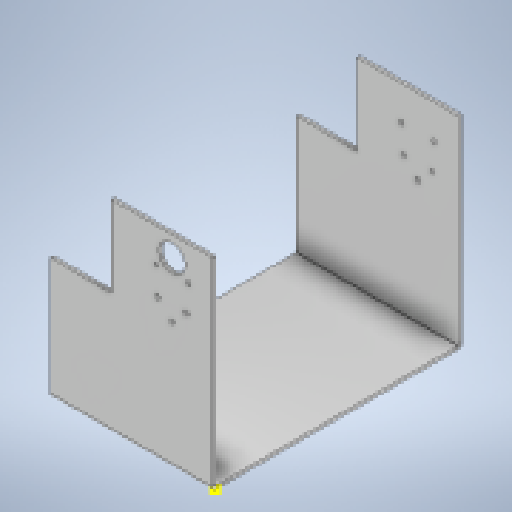
# Autodesk Inventor part: body_main_frame
Saved by Autodesk Inventor 2025.2 (Build 292293000, 293)
## iProperties
Created: 2025-05-07
Part Number: body_main_frame
Material: Aluminum 6061-AHC
Document SubType Name: Sheet Metal
Designer: chris
Density: 2.7 g/cm^3
Sheet Metal Rule: Default_mm
Appearance: Aluminum - Dark
Author: chris
Autodesk Inventor part; units mm, degrees
ref_plane "YZ Plane" through (0, 0, 0) normal (1, 0, 0) x (0, 1, 0)
ref_plane "XZ Plane" through (0, 0, 0) normal (0, 1, 0) x (-1, 0, 0)
ref_plane "XY Plane" through (0, 0, 0) normal (0, 0, 1) x (1, 0, 0)
sketch "Sketch1" plane through (0, 0, 0) normal (0, 1, 0) x (-1, 0, 0)
  line L0 (0, 0) -> (80, 0)
  line L1 (80, 0) -> (80, 120)
  line L2 (80, 120) -> (0, 120)
  line L3 (0, 120) -> (0, 0)
  dimension "d0" = 80
  dimension "d1" = 120
  measures "d0" distance of L2.end L1.end
  measures "d1" distance of L0.end L1.end
extrude "Plate1" add sketch "Sketch1" along normal blind 1.5
sketch "Sketch2" plane through (0, 0, 121.5) normal (0, 0, -1) x (-1, 0, 0)
  line L0 (80, 0) -> (0, 0)
  line L1 (0, 0) -> (0, 100)
  line L2 (0, 100) -> (80, 100)
  line L3 (80, 100) -> (80, 0)
  constraints: 8 end point
edge flange "Flange1" height 100 angle 90 thickness 1.5 bend radius 0.31 thickness toward (0, 0, -1) relief tear relief width 1.5 relief depth 0.75 edges at (-40, 1.5, 120) wall of the first edge with corners at (-80, 0, 121.5) (0, 0, 121.5) (0, 100, 121.5) (-80, 100, 121.5)
bend "Bend1"
corner "Corner1"
sketch "Sketch3" plane through (-80, 0, -1.5) normal (0, 0, 1) x (1, 0, 0)
  line L0 (80, 0) -> (0, 0)
  line L1 (0, 0) -> (0, 100)
  line L2 (0, 100) -> (80, 100)
  line L3 (80, 100) -> (80, 0)
  constraints: 6 end point, 1 horizontal, 1 perpendicular, 1 vertical
edge flange "Flange2" height 100 angle 90 thickness 1.5 bend radius 0.31 thickness toward (0, 0, 1) relief tear relief width 1.5 relief depth 0.75 edges at (-40, 1.5, 0) wall of the first edge with corners at (0, 0, -1.5) (-80, 0, -1.5) (-80, 100, -1.5) (0, 100, -1.5)
bend "Bend2"
corner "Corner2"
sketch "Sketch4" plane through (0, 100, -1.5) normal (0, 0, -1) x (-1, 0, 0)
  line L0 (56, -40) -> (80, -40)
  line L1 (80, -40) -> (80, 0)
  line L2 (80, 0) -> (56, 0)
  line L3 (56, 0) -> (56, -40)
  line L4 (80, 0) -> (80, -98.19) projected
  line L5 (0, 0) -> (80, 0) projected
  point P0 (0, -100)
  dimension "d23" = 24
  dimension "d24" = 40
  constraints: 8 end point, 2 collinear, 2 parallel, 1 horizontal, 1 perpendicular
  measures "d23" distance of L0.start L0.end
  measures "d24" distance of L2.end L0.start
extrude "Cut1" cut sketch "Sketch4" against normal blind 1.5
sketch "Sketch5" plane through (0, 100, 120) normal (0, 0, -1) x (-1, 0, 0)
  point P0 (0, -100)
sketch "Sketch6" plane through (-80, 100, 121.5) normal (0, 0, 1) x (1, 0, 0)
  line L0 (24, 0) -> (0, 0)
  line L1 (0, 0) -> (0, -40)
  line L2 (0, -40) -> (24, -40)
  line L3 (24, -40) -> (24, 0)
  line L4 (0, -98.19) -> (0, 0) projected
  line L5 (0, 0) -> (80, 0) projected
  point P0 (80, -100)
  dimension "d27" = 40
  dimension "d28" = 24
  constraints: 8 end point, 2 collinear, 2 parallel, 1 horizontal, 1 perpendicular
  measures "d27" distance of L2.end L0.start
  measures "d28" distance of L1.end L2.end
extrude "Cut2" cut sketch "Sketch6" against normal blind 1.5
sketch "Sketch7" plane through (0, 1.81, -1.5) normal (0, 0, -1) x (-1, 0, 0)
  circle A0 centre (17.93, 60.77) radius 0.7835 projected
  circle A1 centre (10.93, 68.07) radius 0.7835 projected
  circle A2 centre (24.93, 68.07) radius 0.7835 projected
  circle A3 centre (9.93, 81.29) radius 0.7835 projected
  circle A4 centre (25.93, 81.29) radius 0.7835 projected
  line L0 (24, 59.37) -> (11.86, 59.37) projected
  line L1 (24, 59.37) -> (24, 60.09) projected
  arc A5 (26, 62.09) -> (24, 60.09) centre (26, 60.09) ccw projected
  line L2 (26, 62.09) -> (26.72, 62.09) projected
  line L3 (26.72, 94.19) -> (26.72, 62.09) projected
  line L4 (26.72, 94.19) -> (26, 94.19) projected
  arc A6 (24, 96.19) -> (26, 94.19) centre (26, 96.19) ccw projected
  line L5 (24, 96.19) -> (24, 96.91) projected
  line L6 (11.86, 96.91) -> (24, 96.91) projected
  line L7 (11.86, 96.91) -> (11.86, 96.19) projected
  arc A7 (9.86, 94.19) -> (11.86, 96.19) centre (9.86, 96.19) ccw projected
  line L8 (9.86, 94.19) -> (9.14, 94.19) projected
  line L9 (9.14, 62.09) -> (9.14, 94.19) projected
  line L10 (9.14, 62.09) -> (9.86, 62.09) projected
  arc A8 (11.86, 60.09) -> (9.86, 62.09) centre (9.86, 60.09) ccw projected
  line L11 (11.86, 60.09) -> (11.86, 59.37) projected
  circle A9 centre (17.93, 88.19) radius 6.4 projected
  point P0 (0, -1.81)
  point P1 (11.86, 94.19)
hole "Hole1" at (-10.93, 69.88, -1.5) at (-9.93, 83.1, -1.5) at (-25.93, 83.1, -1.5) at (-24.93, 69.88, -1.5) at (-17.93, 62.58, -1.5) direction (0, 0, 1) diameter 2.1 depth 1.5
sketch "Sketch8" plane through (-80, 1.81, 121.5) normal (0, 0, 1) x (1, 0, 0)
  circle A0 centre (62.07, 60.77) radius 0.7835 projected
  circle A1 centre (55.07, 68.07) radius 0.7835 projected
  circle A2 centre (69.07, 68.07) radius 0.7835 projected
  circle A3 centre (54.07, 81.29) radius 0.7835 projected
  circle A4 centre (70.07, 81.29) radius 0.7835 projected
  line L0 (68.14, 59.37) -> (56, 59.37) projected
  line L1 (68.14, 59.37) -> (68.14, 60.09) projected
  arc A5 (70.14, 62.09) -> (68.14, 60.09) centre (70.14, 60.09) ccw projected
  line L2 (70.14, 62.09) -> (70.86, 62.09) projected
  line L3 (70.86, 94.19) -> (70.86, 62.09) projected
  line L4 (70.86, 94.19) -> (70.14, 94.19) projected
  arc A6 (68.14, 96.19) -> (70.14, 94.19) centre (70.14, 96.19) ccw projected
  line L5 (68.14, 96.19) -> (68.14, 96.91) projected
  line L6 (56, 96.91) -> (68.14, 96.91) projected
  line L7 (56, 96.91) -> (56, 96.19) projected
  arc A7 (54, 94.19) -> (56, 96.19) centre (54, 96.19) ccw projected
  line L8 (54, 94.19) -> (53.28, 94.19) projected
  line L9 (53.28, 62.09) -> (53.28, 94.19) projected
  line L10 (53.28, 62.09) -> (54, 62.09) projected
  arc A8 (56, 60.09) -> (54, 62.09) centre (54, 60.09) ccw projected
  line L11 (56, 60.09) -> (56, 59.37) projected
  circle A9 centre (62.07, 88.19) radius 6.4 projected
  point P0 (80, -1.81)
  point P1 (56, 94.19)
hole "Hole2" at (-25.93, 83.1, 121.5) at (-9.93, 83.1, 121.5) at (-10.93, 69.88, 121.5) at (-24.93, 69.88, 121.5) at (-17.93, 62.58, 121.5) direction (0, 0, -1) diameter 2.1 depth 1.5
sketch "Sketch9" plane through (-80, 1.81, 121.5) normal (0, 0, 1) x (1, 0, 0)
  circle A0 centre (62.07, 60.77) radius 0.7835 projected
  circle A1 centre (55.07, 68.07) radius 0.7835 projected
  circle A2 centre (69.07, 68.07) radius 0.7835 projected
  circle A3 centre (54.07, 81.29) radius 0.7835 projected
  circle A4 centre (70.07, 81.29) radius 0.7835 projected
  line L0 (68.14, 59.37) -> (56, 59.37) projected
  line L1 (68.14, 59.37) -> (68.14, 60.09) projected
  arc A5 (70.14, 62.09) -> (68.14, 60.09) centre (70.14, 60.09) ccw projected
  line L2 (70.14, 62.09) -> (70.86, 62.09) projected
  line L3 (70.86, 94.19) -> (70.86, 62.09) projected
  line L4 (70.86, 94.19) -> (70.14, 94.19) projected
  arc A6 (68.14, 96.19) -> (70.14, 94.19) centre (70.14, 96.19) ccw projected
  line L5 (68.14, 96.19) -> (68.14, 96.91) projected
  line L6 (56, 96.91) -> (68.14, 96.91) projected
  line L7 (56, 96.91) -> (56, 96.19) projected
  arc A7 (54, 94.19) -> (56, 96.19) centre (54, 96.19) ccw projected
  line L8 (54, 94.19) -> (53.28, 94.19) projected
  line L9 (53.28, 62.09) -> (53.28, 94.19) projected
  line L10 (53.28, 62.09) -> (54, 62.09) projected
  arc A8 (56, 60.09) -> (54, 62.09) centre (54, 60.09) ccw projected
  line L11 (56, 60.09) -> (56, 59.37) projected
  circle A9 centre (62.07, 88.19) radius 6.4 projected
  circle A10 centre (62.07, 88.19) radius 6.5
  point P0 (80, -1.81)
  point P1 (56, 94.19)
  dimension "d45" = 13
  constraints: 1 centre point, 1 coincident
  measures "d45" diameter of A10
extrude "Extrusion1" cut sketch "Sketch9" against normal blind 1.5 contours A9 | A10
sketch "Sketch10" plane through (0, 1.81, -1.5) normal (0, 0, -1) x (-1, 0, 0)
  circle A0 centre (17.93, 60.77) radius 0.7835 projected
  circle A1 centre (10.93, 68.07) radius 0.7835 projected
  circle A2 centre (24.93, 68.07) radius 0.7835 projected
  circle A3 centre (9.93, 81.29) radius 0.7835 projected
  circle A4 centre (25.93, 81.29) radius 0.7835 projected
  line L0 (24, 59.37) -> (11.86, 59.37) projected
  line L1 (24, 59.37) -> (24, 60.09) projected
  arc A5 (26, 62.09) -> (24, 60.09) centre (26, 60.09) ccw projected
  line L2 (26, 62.09) -> (26.72, 62.09) projected
  line L3 (26.72, 94.19) -> (26.72, 62.09) projected
  line L4 (26.72, 94.19) -> (26, 94.19) projected
  arc A6 (24, 96.19) -> (26, 94.19) centre (26, 96.19) ccw projected
  line L5 (24, 96.19) -> (24, 96.91) projected
  line L6 (11.86, 96.91) -> (24, 96.91) projected
  line L7 (11.86, 96.91) -> (11.86, 96.19) projected
  arc A7 (9.86, 94.19) -> (11.86, 96.19) centre (9.86, 96.19) ccw projected
  line L8 (9.86, 94.19) -> (9.14, 94.19) projected
  line L9 (9.14, 62.09) -> (9.14, 94.19) projected
  line L10 (9.14, 62.09) -> (9.86, 62.09) projected
  arc A8 (11.86, 60.09) -> (9.86, 62.09) centre (9.86, 60.09) ccw projected
  line L11 (11.86, 60.09) -> (11.86, 59.37) projected
  circle A9 centre (17.93, 88.19) radius 6.4 projected
  circle A10 centre (17.93, 88.19) radius 6.5
  point P0 (0, -1.81)
  point P1 (11.86, 94.19)
  dimension "d48" = 13
  constraints: 1 centre point, 1 coincident
  measures "d48" diameter of A10
extrude "Extrusion2" cut sketch "Sketch10" against normal blind 1.5 contours A9 | A10
equation "\"d25\" = Thickness"
equation "\"d29\" = Thickness"
equation "\"d36\" = Thickness"
equation "\"d43\" = Thickness"
equation "\"d2\" = Thickness"
equation "\"d3\" = BendReliefWidth"
equation "\"d4\" = BendReliefDepth"
equation "\"d5\" = MinimumRemnant"
equation "\"d6\" = TransitionRadius"
equation "\"d9\" = BendRadius"
equation "\"d10\" = CornerReliefSize"
equation "\"d11\" = GapSize"
equation "\"d12\" = JacobiRadiusSize"
equation "\"d13\" = BendReliefWidth"
equation "\"d14\" = BendReliefDepth"
equation "\"d15\" = MinimumRemnant"
equation "\"d16\" = TransitionRadius"
equation "\"d19\" = BendRadius"
equation "\"d20\" = CornerReliefSize"
equation "\"d21\" = GapSize"
equation "\"d22\" = JacobiRadiusSize"
equation "\"BendReliefWidth\" = Thickness"
equation "\"BendReliefDepth\" = 0.5 * Thickness"
equation "\"CornerReliefSize\" = 4 * Thickness"
equation "\"MinimumRemnant\" = 2 * Thickness"
equation "\"TransitionRadius\" = BendRadius"
equation "\"JacobiRadiusSize\" = BendRadius"
equation "\"GapSize\" = Thickness"
equation "\"Thickness\" = 1.5"
equation "\"BendRadius\" = 0.31"
body "Solid1"
